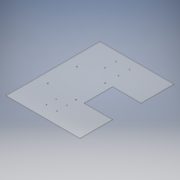
# Autodesk Inventor part: Small Wall
Saved by Autodesk Inventor 2017 (Build 210142000, 142)
## iProperties
Created: 2020-02-08
Part Number: Small Wall
Material: Polycarbonate, Clear
Document SubType Name: Modeling
Designer: S347041956
Density: 1.2 g/cm^3
Appearance: Polycarbonate - Clear
Author: S347041956
Autodesk Inventor part; units mm, degrees
ref_plane "YZ Plane" through (0, 0, 0) normal (1, 0, 0) x (0, 1, 0)
ref_plane "XZ Plane" through (0, 0, 0) normal (0, 1, 0) x (-1, 0, 0)
ref_plane "XY Plane" through (0, 0, 0) normal (0, 0, 1) x (1, 0, 0)
sketch "Sketch1" plane through (0, 0, 0) normal (1, 0, 0) x (0, 1, 0)
  line L0 (1.2792, 416.4647) -> (-1.2608, 416.4647)
  line L1 (-1.2608, 416.4647) -> (-1.2608, -2.6353)
  line L2 (-1.2608, -2.6353) -> (1.2792, -2.6353)
  line L3 (1.2792, -2.6353) -> (1.2792, 416.4647)
  point P0 (0, 0)
  dimension "d0" = 2.54
  dimension "d1" = 419.1
  constraints: 8 end point, 2 parallel, 1 horizontal, 1 perpendicular
  measures "d0" distance between parallel lines of L1 L3
  measures "d1" distance between parallel lines of L2 L0
extrude "Extrusion1" add sketch "Sketch1" along normal blind 330.2
sketch "Sketch2" plane through (0, -1.2608, -2.6353) normal (0, -1, 0) x (1, 0, 0)
  circle A0 centre (173.4912, 364.1066) radius 1.8317
  circle A1 centre (173.4912, 321.15) radius 1.8569
  circle A2 centre (125.7136, 321.15) radius 1.6798
  circle A3 centre (125.7136, 364.1066) radius 1.8317
  circle A4 centre (172.0099, 278.3905) radius 2.4145
  circle A5 centre (172.0099, 149.0149) radius 2.2543
  circle A6 centre (45.2863, 149.0149) radius 2.2807
  circle A7 centre (45.2863, 278.3905) radius 2.4145
  circle A8 centre (173.7693, 90.9127) radius 1.8262
  circle A9 centre (173.7693, 42.0819) radius 1.8081
  circle A10 centre (112.7456, 42.0819) radius 1.7821
  circle A11 centre (112.7456, 90.9127) radius 1.8323
  point P0 (0, 2.6353)
  constraints: 12 centre point
extrude "Extrusion2" cut sketch "Sketch2" against normal up to surface (2.54 mm away)
sketch "Sketch3" plane through (0, 1.2792, 416.4647) normal (0, 1, 0) x (1, 0, 0)
  line L0 (266.7, 209.1248) -> (266.7, 419.1) construction
  line L1 (0, 419.1) -> (330.2, 419.1) projected
  line L2 (266.7, 209.1248) -> (266.7, -0.8504) construction
  line L3 (330.2, 0) -> (330.2, 419.1) projected
  line L4 (330.2, 272.4308) -> (203.2, 272.4308)
  line L5 (203.2, 272.4308) -> (203.2, 145.4308)
  line L6 (203.2, 145.4308) -> (330.2, 145.4308)
  line L7 (330.2, 145.4308) -> (330.2, 272.4308)
  line L8 (330.2, 208.9308) -> (203.2, 208.9308) construction
  point P0 (0, 416.4647)
  dimension "d10" = 127
  dimension "d11" = 127
  dimension "d12" = 63.5
  constraints: 14 end point, 3 point on line, 2 midpoint, 2 parallel, 1 collinear, 1 horizontal, 1 perpendicular, 1 vertical
  measures "d10" distance of L6.end L5.end
  measures "d11" distance of L5.end L4.end
  measures "d12" distance between parallel lines of L3 L0
extrude "Extrusion4" cut sketch "Sketch3" against normal up to surface (2.54 mm away)
body "Solid1"
